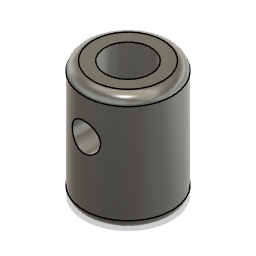
Circular_Support (Autodesk Fusion 360 archive; units mm, degrees)
design "Spacer"
Autodesk Fusion 360 part; units mm, degrees
sketch "Sketch1" plane through (0, 0, 0) normal (0, 1, 0) x (1, 0, 0)
  circle A0 centre (150, 0) radius 4.95
  circle A1 centre (150, 0) radius 2.575
  dimension "d1" = 9.9
  dimension "d2" = 5.15
  constraint concentric A0 A1
  measures "d1" diameter of A0
  measures "d2" diameter of A1
extrude "Extrude1" add sketch "Sketch1" along normal blind 13.15
ref_plane "WorkPlane1" through (150, 7.9424, 4.95) normal (0, 0, 1) x (-1, 0, 0)
sketch "Sketch2" plane through (0, 0, 4.95) normal (0, 0, 1) x (1, 0, 0)
  line L0 (154.95, 13.15) -> (145.05, 13.15) construction
  line L1 (154.95, 0) -> (145.05, 0) construction
  line L2 (150, 13.15) -> (150, 0) construction
  circle A0 centre (150, 8.15) radius 1.6
  dimension "d6" = 3.2
  dimension "d7" = 5
  constraint midpoint L0 L2.start
  constraint midpoint L1 L2.end
  constraint coincident L2 A0.centre
  measures "d6" diameter of A0
  measures "d7" distance of L0 A0.centre
extrude "Extrude2" cut sketch "Sketch2" against normal blind 16
fillet "Fillet1" radius 1 2 edges at (145.385, 13.15, 1.79) (145.385, 0, 1.79)
